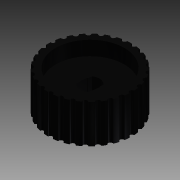
# Autodesk Inventor part: Llave hornillo
Saved by Autodesk Inventor 2014 (Build 180170000, 170)
## iProperties
Created: 2017-05-23
Part Number: Llave hornillo
Material: Generic
Document SubType Name: Modeling
Designer: resaj
Density: 1 g/cm^3
Appearance: Smooth - Black
Author: resaj
Autodesk Inventor part; units mm, degrees
ref_plane "YZ Plane" through (0, 0, 0) normal (1, 0, 0) x (0, 1, 0)
ref_plane "XZ Plane" through (0, 0, 0) normal (0, 1, 0) x (-1, 0, 0)
ref_plane "XY Plane" through (0, 0, 0) normal (0, 0, 1) x (1, 0, 0)
sketch "Sketch1" plane through (0, 0, 0) normal (0, 1, 0) x (-1, 0, 0)
  circle A0 centre (0, 0) radius 18.5
  dimension "d0" = 37
  constraints: 1 centre point, 1 coincident
  measures "d0" diameter of A0
extrude "Extrusion1" add sketch "Sketch1" along normal blind 17
sketch "Sketch2" plane through (0, 17, 0) normal (0, 1, 0) x (1, 0, 0)
  circle A0 centre (0, 0) radius 18.5 projected
  circle A1 centre (18.5, 0) radius 1
  line L0 (0, 0) -> (18.5, 0) construction
  dimension "d3" = 2
  constraints: 2 end point, 1 centre point, 1 horizontal, 1 horizontal alignment, 1 other
  measures "d3" diameter of A1
extrude "Extrusion2" cut sketch "Sketch2" against normal through all contours A0 A1 | A0 A1 picked at (18.1866, 0.2274) picked at (18.7982, 0.2581)
pattern_circular "Circular Pattern1" count 29 over 360 about axis through (0, 0, 0) along (0, 1, 0) of "Extrusion2"
sketch "Sketch3" plane through (0, 0, 0) normal (0, -1, 0) x (1, 0, 0)
  arc A0 (17.8262, 4.9474) -> (17.1854, 6.8494) centre (0, 0) ccw projected
hole "Hole1" at (0, 0, 0) direction (0, 1, 0) diameter 3.5 end through all countersink diameter 9.5 countersink angle 90
sketch "Sketch4" plane through (0, 0, 0) normal (0, -1, 0) x (1, 0, 0)
  circle A0 centre (0, 0) radius 4.75 projected
  arc A1 (-18.4728, 1.0035) -> (-18.4728, -1.0035) centre (0, 0) ccw projected
  arc A2 (18.473, 0.9996) -> (18.256, 2.9949) centre (0, 0) ccw projected
  line L0 (-14.75, 1.25) -> (-6.75, 1.25)
  line L1 (-6.75, 1.25) -> (-6.75, -1.25)
  line L2 (-6.75, -1.25) -> (-14.75, -1.25)
  line L3 (-14.75, -1.25) -> (-14.75, 1.25)
  line L4 (-18.5, 0) -> (0, 0) construction
  line L5 (-10.75, 1.25) -> (-10.75, 0) construction
  line L6 (-10.75, 0) -> (-10.75, -1.25) construction
  circle A3 centre (0, 0) radius 11.4692 construction
  line L7 (-0.2594, 7.791) -> (2.8062, 7.791) construction
  line L8 (2.8062, 7.791) -> (2.8062, 10.4034) construction
  line L9 (2.8062, 10.4034) -> (0.8969, 11.8689) construction
  line L10 (0.8969, 11.8689) -> (0.2634, 13.3204) construction
  line L11 (0.2634, 13.3204) -> (-0.0505, 15.6348) construction
  spline S0 degree 4 poles (-0.2594, 7.791) (2.8062, 7.791) (2.8062, 10.4034) (0.8969, 11.8689) (0.2634, 13.3204) (-0.0505, 15.6348) knots 1 1 1 1 1 2 3 3 3 3 3
  line L12 (-0.2594, 7.791) -> (-3.3031, 7.791) construction
  line L13 (-3.3031, 7.791) -> (-4.0256, 9.1624) construction
  line L14 (-4.0256, 9.1624) -> (-3.2524, 11.7471) construction
  spline S1 degree 3 poles (-0.2594, 7.791) (-3.3031, 7.791) (-4.0256, 9.1624) (-3.2524, 11.7471) knots 1 1 1 1 2 2 2 2
  line L15 (-3.2524, 11.7471) -> (-2.5295, 10.0909) construction
  line L16 (-2.5295, 10.0909) -> (-2.3206, 10.0909) construction
  line L17 (-2.3206, 10.0909) -> (-2.3206, 12.6773) construction
  line L18 (-2.3206, 12.6773) -> (-0.0505, 15.6348) construction
  spline S2 degree 4 poles (-3.2524, 11.7471) (-2.5295, 10.0909) (-2.3206, 10.0909) (-2.3206, 12.6773) (-0.0505, 15.6348) knots 1 1 1 1 1 2 2 2 2 2
  line L19 (5.6325, 5.7441) -> (6.9202, 4.4564) construction
  line L20 (6.9202, 4.4564) -> (8.0174, 5.5537) construction
  line L21 (8.0174, 5.5537) -> (7.8311, 6.9712) construction
  line L22 (7.8311, 6.9712) -> (8.1746, 7.8469) construction
  line L23 (8.1746, 7.8469) -> (9.0149, 8.9509) construction
  spline S3 degree 4 poles (5.6325, 5.7441) (6.9202, 4.4564) (8.0174, 5.5537) (7.8311, 6.9712) (8.1746, 7.8469) (9.0149, 8.9509) knots 1 1 1 1 1 2 3 3 3 3 3
  line L24 (5.6325, 5.7441) -> (4.354, 7.0226) construction
  line L25 (4.354, 7.0226) -> (4.6267, 7.9019) construction
  line L26 (4.6267, 7.9019) -> (6.0371, 8.6628) construction
  spline S4 degree 3 poles (5.6325, 5.7441) (4.354, 7.0226) (4.6267, 7.9019) (6.0371, 8.6628) knots 1 1 1 1 2 2 2 2
  line L27 (6.0371, 8.6628) -> (5.6451, 7.6636) construction
  line L28 (5.6451, 7.6636) -> (5.7328, 7.5758) construction
  line L29 (5.7328, 7.5758) -> (6.8191, 8.6622) construction
  line L30 (6.8191, 8.6622) -> (9.0149, 8.9509) construction
  spline S5 degree 4 poles (6.0371, 8.6628) (5.6451, 7.6636) (5.7328, 7.5758) (6.8191, 8.6622) (9.0149, 8.9509) knots 1 1 1 1 1 2 2 2 2 2
  arc A4 (18.256, -2.9949) -> (18.473, -0.9996) centre (0, 0) ccw projected
  line L31 (0, 0) -> (13.0815, 13.0815) construction
  line L32 (0, 0) -> (18.5, 0) construction
  dimension "d16" = 2.5
  dimension "d17" = 8
  dimension "d18" = 2
  dimension "d21" = 0.7224
  dimension "d23" = 2.5841
  dimension "d24" = 0.6335
  dimension "d25" = 1.9093
  dimension "d26" = 1.3714
  dimension "d27" = 0.9285
  dimension "d28" = 0.3125
  dimension "d30" = 0.8084
  dimension "d31" = 0.6431
  dimension "d32" = 2.3144
  dimension "d33" = 1.3437
  dimension "d34" = 0.1218
  dimension "d48" = 0.0508
  dimension "d50" = 0.2089
  dimension "d81" = 45
  constraints: 18 end point, 8 parallel, 5 perpendicular, 2 equal length, 2 horizontal, 2 midpoint, 2 point on circle, 1 centre point, 1 coincident, 1 point on line, 1 vertical, 18 other
  measures "d16" distance of L0.end L1.end
  measures "d17" distance of L0.start L0.end
  measures "d18" distance edge to line of A0 L1
  measures "d21" horizontal distance of L12.end L13.end
  measures "d23" horizontal distance of L10.end L16.end
  measures "d24" horizontal distance of L9.end L10.end
  measures "d25" horizontal distance of L7.end L9.end
  measures "d26" vertical distance of L13.end L12.end
  measures "d27" vertical distance of L16.end L13.end
  measures "d28" vertical distance of L8.end L16.end
  measures "d30" vertical distance of L17.end L9.end
  measures "d31" vertical distance of L10.end L17.end
  measures "d32" vertical distance of L11.end L10.end
  measures "d33" vertical distance of L14.end L8.end
  measures "d34" vertical distance of L9.end L14.end
  measures "d48" horizontal distance of L14.end L12.end
  measures "d50" distance of L15.end L16.end
  measures "d81" angle of L32 L31
extrude "Extrusion3" cut sketch "Sketch4" against normal blind 1 contours L0 L1 L2 L3 | S1 S2 S0 | S4 S5 S3
sketch "Sketch5" plane through (0, 17, 0) normal (0, 1, 0) x (1, 0, 0)
  circle A0 centre (0, 0) radius 1.75 projected
  arc A1 (17.1854, -6.8494) -> (17.8262, -4.9474) centre (0, 0) ccw projected
  circle A2 centre (0, 0) radius 15.15
  dimension "d82" = 30.3
  constraints: 1 centre point, 1 coincident
  measures "d82" diameter of A2
extrude "Extrusion4" cut sketch "Sketch5" against normal blind 6.25
sketch "Sketch6" plane through (0, 10.75, 0) normal (0, 1, 0) x (1, 0, 0)
  circle A0 centre (0, 0) radius 1.75 projected
  circle A1 centre (0, 0) radius 15.15 projected
  circle A2 centre (0, 0) radius 4.2
  line L0 (-2.5001, 3.3748) -> (-2.6767, 1.7494)
  line L1 (3.1666, 2.7592) -> (2.9899, 1.1337)
  line L2 (-2.5001, 3.3748) -> (3.1666, 2.7592) construction
  line L3 (-2.6767, 1.7494) -> (-2.9749, 1.7818)
  line L4 (-2.9749, 1.7818) -> (-3.2882, -1.1013)
  line L5 (-3.2882, -1.1013) -> (-2.9899, -1.1337)
  line L6 (-2.9899, -1.1337) -> (2.6767, -1.7494) construction
  line L7 (-2.6767, 1.7494) -> (2.9899, 1.1337) construction
  line L8 (2.9899, 1.1337) -> (3.2882, 1.1013)
  line L9 (3.2882, 1.1013) -> (2.9749, -1.7818)
  line L10 (2.9749, -1.7818) -> (2.6767, -1.7494)
  line L11 (-3.1316, 0.3402) -> (0, 0) construction
  line L12 (-2.9899, -1.1337) -> (-3.1666, -2.7592)
  line L13 (-2.6767, 1.7494) -> (-2.9899, -1.1337) construction
  line L14 (2.9899, 1.1337) -> (2.6767, -1.7494) construction
  line L15 (2.6767, -1.7494) -> (2.5001, -3.3748)
  circle A3 centre (0, 0) radius 15.15 construction
  arc A4 (18.256, -2.9949) -> (17.8262, -4.9474) centre (18.0675, -3.977) ccw construction
  arc A5 (18.256, -2.9949) -> (18.473, -0.9996) centre (0, 0) ccw construction
  arc A6 (18.473, 0.9996) -> (18.473, -0.9996) centre (18.5, 0) ccw construction
  arc A7 (18.473, 0.9996) -> (18.256, 2.9949) centre (0, 0) ccw construction
  arc A8 (17.8262, 4.9474) -> (18.256, 2.9949) centre (18.0675, 3.977) ccw construction
  arc A9 (17.8262, 4.9474) -> (17.1854, 6.8494) centre (0, 0) ccw construction
  arc A10 (16.3459, 8.6638) -> (17.1854, 6.8494) centre (16.7901, 7.7679) ccw construction
  arc A11 (16.3459, 8.6638) -> (15.3112, 10.3836) centre (0, 0) ccw construction
  arc A12 (14.1013, 11.9752) -> (15.3112, 10.3836) centre (14.7277, 11.1957) ccw construction
  arc A13 (14.1013, 11.9752) -> (12.721, 13.4322) centre (0, 0) ccw construction
  arc A14 (11.1973, 14.7265) -> (12.721, 13.4322) centre (11.9766, 14.1) ccw construction
  arc A15 (11.1973, 14.7265) -> (9.5361, 15.8529) centre (0, 0) ccw construction
  arc A16 (7.7697, 16.7893) -> (9.5361, 15.8529) centre (8.6656, 16.345) ccw construction
  arc A17 (7.7697, 16.7893) -> (5.9052, 17.5322) centre (0, 0) ccw construction
  arc A18 (3.9788, 18.0671) -> (5.9052, 17.5322) centre (4.9493, 17.8257) ccw construction
  arc A19 (3.9788, 18.0671) -> (1.9983, 18.3918) centre (0, 0) ccw construction
  arc A20 (0.0019, 18.5) -> (1.9983, 18.3918) centre (1.0016, 18.4729) ccw construction
  arc A21 (0.0019, 18.5) -> (-2.0021, 18.3913) centre (0, 0) ccw construction
  arc A22 (-3.9751, 18.0679) -> (-2.0021, 18.3913) centre (-2.993, 18.2563) ccw construction
  arc A23 (-3.9751, 18.0679) -> (-5.9089, 17.531) centre (0, 0) ccw construction
  arc A24 (-7.7662, 16.791) -> (-5.9089, 17.531) centre (-6.8476, 17.1861) ccw construction
  arc A25 (-7.7662, 16.791) -> (-9.5394, 15.8509) centre (0, 0) ccw construction
  arc A26 (-11.1942, 14.7289) -> (-9.5394, 15.8509) centre (-10.382, 15.3122) ccw construction
  arc A27 (-11.1942, 14.7289) -> (-12.7238, 13.4296) centre (0, 0) ccw construction
  arc A28 (-14.0987, 11.9781) -> (-12.7238, 13.4296) centre (-13.4309, 12.7224) ccw construction
  arc A29 (-14.0987, 11.9781) -> (-15.3133, 10.3804) centre (0, 0) ccw construction
  arc A30 (-16.3441, 8.6673) -> (-15.3133, 10.3804) centre (-15.8519, 9.5377) ccw construction
  arc A31 (-16.3441, 8.6673) -> (-17.1868, 6.8458) centre (0, 0) ccw construction
  arc A32 (-17.8252, 4.9511) -> (-17.1868, 6.8458) centre (-17.5316, 5.9071) ccw construction
  arc A33 (-17.8252, 4.9511) -> (-18.2566, 2.9911) centre (0, 0) ccw construction
  arc A34 (-18.4728, 1.0035) -> (-18.2566, 2.9911) centre (-18.3916, 2.0002) ccw construction
  arc A35 (-18.4728, 1.0035) -> (-18.4728, -1.0035) centre (0, 0) ccw construction
  arc A36 (-18.2566, -2.9911) -> (-18.4728, -1.0035) centre (-18.3916, -2.0002) ccw construction
  arc A37 (-18.2566, -2.9911) -> (-17.8252, -4.9511) centre (0, 0) ccw construction
  arc A38 (-17.1868, -6.8458) -> (-17.8252, -4.9511) centre (-17.5316, -5.9071) ccw construction
  arc A39 (-17.1868, -6.8458) -> (-16.3441, -8.6673) centre (0, 0) ccw construction
  arc A40 (-15.3133, -10.3804) -> (-16.3441, -8.6673) centre (-15.8519, -9.5377) ccw construction
  arc A41 (-15.3133, -10.3804) -> (-14.0987, -11.9781) centre (0, 0) ccw construction
  arc A42 (-12.7238, -13.4296) -> (-14.0987, -11.9781) centre (-13.4309, -12.7224) ccw construction
  arc A43 (-12.7238, -13.4296) -> (-11.1942, -14.7289) centre (0, 0) ccw construction
  arc A44 (-9.5394, -15.8509) -> (-11.1942, -14.7289) centre (-10.382, -15.3122) ccw construction
  arc A45 (-9.5394, -15.8509) -> (-7.7662, -16.791) centre (0, 0) ccw construction
  arc A46 (-5.9089, -17.531) -> (-7.7662, -16.791) centre (-6.8476, -17.1861) ccw construction
  arc A47 (-5.9089, -17.531) -> (-3.9751, -18.0679) centre (0, 0) ccw construction
  arc A48 (-2.0021, -18.3913) -> (-3.9751, -18.0679) centre (-2.993, -18.2563) ccw construction
  arc A49 (-2.0021, -18.3913) -> (0.0019, -18.5) centre (0, 0) ccw construction
  arc A50 (1.9983, -18.3918) -> (0.0019, -18.5) centre (1.0016, -18.4729) ccw construction
  arc A51 (1.9983, -18.3918) -> (3.9788, -18.0671) centre (0, 0) ccw construction
  arc A52 (5.9052, -17.5322) -> (3.9788, -18.0671) centre (4.9493, -17.8257) ccw construction
  arc A53 (5.9052, -17.5322) -> (7.7697, -16.7893) centre (0, 0) ccw construction
  arc A54 (9.5361, -15.8529) -> (7.7697, -16.7893) centre (8.6656, -16.345) ccw construction
  arc A55 (9.5361, -15.8529) -> (11.1973, -14.7265) centre (0, 0) ccw construction
  arc A56 (12.721, -13.4322) -> (11.1973, -14.7265) centre (11.9766, -14.1) ccw construction
  arc A57 (12.721, -13.4322) -> (14.1013, -11.9752) centre (0, 0) ccw construction
  arc A58 (15.3112, -10.3836) -> (14.1013, -11.9752) centre (14.7277, -11.1957) ccw construction
  arc A59 (15.3112, -10.3836) -> (16.3459, -8.6638) centre (0, 0) ccw construction
  arc A60 (17.1854, -6.8494) -> (16.3459, -8.6638) centre (16.7901, -7.7679) ccw construction
  arc A61 (17.1854, -6.8494) -> (17.8262, -4.9474) centre (0, 0) ccw construction
  line L16 (1.9983, 18.3918) -> (0, 0) construction
  dimension "d85" = 8.4
  dimension "d86" = 5.7
  dimension "d87" = 2.9
  dimension "d88" = 6.3
  constraints: 34 end point, 18 parallel, 15 perpendicular, 4 point on circle, 2 collinear, 1 centre point, 1 coincident, 1 midpoint, 1 point on line
  measures "d85" diameter of A2
  measures "d86" distance between parallel lines of L1 L0
  measures "d87" distance of L3.end L4.end
  measures "d88" distance between parallel lines of L9 L4
extrude "Extrusion5" cut sketch "Sketch6" against normal blind 5.5 contours L1 L8 L9 L10 L15 A2 L12 L5 L4 L3 L0
body "Solid1"
